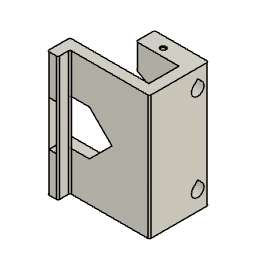
Ryobi PCL424 Cordless Trim Router Adjustable Fence (Autodesk Fusion 360 design; units mm, degrees)
Autodesk Fusion 360 part; units mm, degrees
sketch "Sketch1" plane through (0, 0, 0) normal (1, 0, 0) x (0, 1, 0)
  line L0 (0, 0) -> (29.2, 0) construction
  circle A0 centre (29.2, 0) radius 4.2
  line L1 (0, 2.5) -> (0, 20) construction
  circle A1 centre (-29.2, 0) radius 4.2
  line L2 (-29.2, 0) -> (-29.2, -4.2) construction
  line L3 (36.4, -5.2) -> (36.4, 7.2)
  line L4 (-36.4, -5.2) -> (-36.4, 7.2)
  line L5 (36.4, -5.2) -> (-36.4, -5.2)
  line L6 (36.4, 7.2) -> (-36.4, 7.2)
  line L7 (29.2, 0) -> (29.2, -4.2) construction
  line L8 (29.2, 0) -> (33.4, 0) construction
  line L9 (29.2, 0) -> (29.2, 4.2) construction
  dimension "d1" = 8.4
  dimension "d2" = 58.4
  dimension "d5" = 1
  dimension "d7" = 3
  dimension "d8" = 3
  constraint coincident L0.start origin
  constraint horizontal L0
  constraint coincident L0.end A0.centre
  constraint symmetric A0 L1 A1
  constraint coincident A1.centre L2.start
  constraint coincident A1 L2.end
  constraint vertical L3
  constraint symmetric L1 L3.start L4.start
  constraint symmetric L1 L3.end L4.end
  constraint coincident A0 L7.end
  constraint perpendicular L0 L7
  constraint coincident A0 L8.end
  constraint perpendicular L7 L8
  constraint coincident A0 L9.end
  constraint perpendicular L8 L9
  measures "d1" diameter of A0
  measures "d2" distance of L0.end A1.centre
  measures "d5" distance of L5 L7.end
  measures "d7" distance of L3 L8.end
  measures "d8" distance of L6 L9.end
extrude "Extrude1" add sketch "Sketch1" along normal blind 36
sketch "Sketch2" plane through (0, 0, -5.2) normal (0, 0, -1) x (1, 0, 0)
  line L0 (0, 36.4) -> (0, -36.4)
  line L1 (0, -36.4) -> (36, -36.4)
  line L2 (36, -36.4) -> (36, 36.4)
  line L3 (36, 36.4) -> (0, 36.4)
  line L4 (0, 0) -> (36, 0) construction
  line L5 (0, 0) -> (-9, 0) construction
  arc A0 (0, -24.9249) -> (0, 24.9249) centre (-9, 0) ccw
  line L6 (0, 36.4) -> (36, 36.4)
  line L7 (0, -36.4) -> (0, 36.4)
  line L8 (36, -36.4) -> (36, 36.4)
  line L9 (0, -36.4) -> (36, -36.4)
  arc A1 (0, -37.9473) -> (0, 37.9473) centre (-9, 0) ccw
  line L10 (28.7, -9.9855) -> (28.7, -36.4)
  line L11 (28.7, 9.9855) -> (28.7, 36.4)
  line L12 (28.7, 9.9855) -> (28.7, -9.9855)
  dimension "d11" = 45
  dimension "d12" = 53
  dimension "d15" = 39
  dimension "d29" = 7.3
  constraint coincident L4.start L5.start
  constraint midpoint L2 L4.end
  constraint perpendicular L0 L5
  constraint coincident L5.end A0.centre
  constraint coincident L0 A0.end
  constraint coincident L0 A0.start
  constraint coincident L7 A1.start
  constraint coincident L7 A1.end
  constraint coincident A1 L10.start
  constraint symmetric L4 L10.start L11.start
  constraint coincident L9 L10.end
  constraint perpendicular L9 L10
  constraint coincident L6 L11.end
  constraint perpendicular L6 L11
  measures "d11" distance of L4.end L5.end
  measures "d12" diameter of A0
  measures "d15" radius of A1
  measures "d29" distance of L2.end L11.end
extrude "Extrude2" cut sketch "Sketch2" against normal up to surface (12.4 mm away) contours L0 A0 L7
extrude "Extrude3" add sketch "Sketch2" along normal blind 20 contours L1 L2 L3 L6 L8 L9 A1 L10 L11 | A1 L12
sketch "Sketch4" plane through (0, 0, -25.2) normal (0, 0, -1) x (1, 0, 0)
  line L0 (28.7, 36.4) -> (28.7, -36.4)
  line L1 (28.7, -36.4) -> (36, -36.4)
  line L2 (36, -36.4) -> (36, 36.4)
  line L3 (36, 36.4) -> (28.7, 36.4)
  line L4 (36, -36.4) -> (-24, -36.4)
  line L5 (-24, -36.4) -> (-24, 36.4)
  line L6 (-24, 36.4) -> (36, 36.4)
  line L7 (36, 36.4) -> (36, -36.4)
  dimension "d30" = 60
  constraint horizontal L4
  constraint vertical L5
  constraint horizontal L6
  constraint vertical L7
  constraint coincident L1.end L2.start
  measures "d30" distance of L1.end L4.end
extrude "Extrude5" add sketch "Sketch4" along normal blind 15
sketch "Sketch5" plane through (0, -36.4, 0) normal (0, -1, 0) x (1, 0, 0)
  line L0 (0, 7.2) -> (0, -5.2)
  line L1 (0, -5.2) -> (28.7, -5.2)
  line L2 (28.7, -5.2) -> (28.7, -25.2)
  line L3 (28.7, -25.2) -> (-24, -25.2)
  line L4 (-24, -25.2) -> (-24, -40.2)
  line L5 (-24, -40.2) -> (36, -40.2)
  line L6 (36, -40.2) -> (36, 7.2)
  line L7 (36, 7.2) -> (0, 7.2)
  line L8 (36, -40.2) -> (-17, -40.2)
  line L9 (-17, -40.2) -> (-17, -32.2)
  line L10 (-17, -32.2) -> (36, -32.2)
  line L11 (36, -32.2) -> (36, -40.2)
  dimension "d33" = 7
  dimension "d34" = 7
  constraint horizontal L8
  constraint vertical L9
  constraint horizontal L10
  constraint vertical L11
  constraint coincident L5.end L6.start
  measures "d33" distance of L3 L10
  measures "d34" distance of L4 L9
extrude "Extrude6" cut sketch "Sketch5" against normal blind 72.8 contours L5 L6 L8 L9 L10 L11
sketch "Sketch6" plane through (0, 0, -32.2) normal (0, 0, -1) x (1, 0, 0)
  line L0 (36, 36.4) -> (-17, 36.4)
  line L1 (-17, 36.4) -> (-17, -36.4)
  line L2 (-17, -36.4) -> (36, -36.4)
  line L3 (36, -36.4) -> (36, 36.4)
  line L4 (-24, 36.4) -> (-24, -36.4)
  line L5 (-24, 15) -> (-4, 15)
  line L6 (-4, 15) -> (11, 0)
  line L7 (1.75, 0) -> (22.5, 0)
  line L8 (-4, -15) -> (11, 0)
  line L9 (-24, -15) -> (-4, -15)
  dimension "d37" = 30
  dimension "d38" = 35
  constraint coincident L4 L5.start
  constraint perpendicular L4 L5
  constraint symmetric L5.start L7 L9.start
  constraint symmetric L5.end L7 L8.start
  constraint symmetric L6.end L7 L8.end
  constraint perpendicular L6 L8
  constraint coincident L6.end L7
  measures "d37" distance of L5 L9
  measures "d38" distance of L4 L6.end
extrude "Extrude7" cut sketch "Sketch6" along normal blind 8 and the other way blind 7 contours L1 L5 L6 L8 L9 | L1 L4 L5 L9
move_face "OffsetFaces1" offset 5 2 faces at (21.5667, 36.4, 3.0667) (21.5667, -36.4, 3.0667)
sketch "Sketch7" plane through (0, 41.4, 0) normal (0, 1, 0) x (-1, 0, 0)
  line L0 (-36, -32.2) -> (17, -32.2)
  line L1 (17, -32.2) -> (17, -40.2)
  line L2 (17, -40.2) -> (24, -40.2)
  line L3 (24, -40.2) -> (24, -25.2)
  line L4 (24, -25.2) -> (-28.7, -25.2)
  line L5 (-28.7, -25.2) -> (-28.7, -5.2)
  line L6 (-28.7, -5.2) -> (0, -5.2)
  line L7 (0, -5.2) -> (0, 7.2)
  line L8 (0, 7.2) -> (-36, 7.2)
  line L9 (-36, 7.2) -> (-36, -32.2)
  circle A0 centre (-13, 0) radius 1.35
  line L10 (0, -4.2) -> (0, 4.2)
  line L11 (0, 0) -> (-13, 0) construction
  dimension "d44" = 2.7
  dimension "d47" = 13
  constraint coincident L11.start origin
  constraint coincident A0.centre L11.end
  constraint horizontal L11
  measures "d44" diameter of A0
  measures "d47" distance of L7 A0.centre
extrude "Extrude8" cut sketch "Sketch7" against normal blind 10 contours A0
mirror "Mirror1" about plane through (0, 0, 0) normal (0, 1, 0) of "Extrude8"
fillet "Fillet4" radius 1 14 edges at (36, 0, -32.2) (-17, -28.2, -32.2) (-17, -28.2, -40.2) (-17, 28.2, -32.2) (-17, 28.2, -40.2) (36, 0, 7.2) (0, -33.1624, 7.2) (0, 33.1624, 7.2) (0, 33.1624, -5.2) (0, -33.1624, -5.2) (-24, -28.2, -40.2) (-24, 28.2, -40.2) (-24, 28.2, -25.2) (-24, -28.2, -25.2)
sketch "Support Material" plane through (0, -15, 0) normal (0, 1, 0) x (-1, 0, 0)
  arc A0 (24, -26.2) -> (23, -25.2) centre (23, -26.2) ccw
  line L0 (23, -25.2) -> (4, -25.2)
  line L1 (4, -25.2) -> (4, -32.2)
  line L2 (4, -32.2) -> (16, -32.2)
  arc A1 (17, -33.2) -> (16, -32.2) centre (16, -33.2) ccw
  line L3 (17, -33.2) -> (17, -39.2)
  arc A2 (17, -39.2) -> (18, -40.2) centre (18, -39.2) ccw
  line L4 (18, -40.2) -> (23, -40.2)
  arc A3 (23, -40.2) -> (24, -39.2) centre (23, -39.2) ccw
  line L5 (24, -39.2) -> (24, -26.2)
  circle A4 centre (-13, 0) radius 1.35
  arc A5 (24, -26.2) -> (23, -25.2) centre (23, -26.2) ccw
  line L6 (24, -26.2) -> (24, -39.2)
  arc A6 (23, -40.2) -> (24, -39.2) centre (23, -39.2) ccw
  line L7 (23, -40.2) -> (18, -40.2)
  arc A7 (17, -39.2) -> (18, -40.2) centre (18, -39.2) ccw
  line L8 (17, -39.2) -> (17, -33.2)
  arc A8 (17, -33.2) -> (16, -32.2) centre (16, -33.2) ccw
  line L9 (16, -32.2) -> (-35, -32.2)
  arc A9 (-36, -31.2) -> (-35, -32.2) centre (-35, -31.2) ccw
  line L10 (-36, -31.2) -> (-36, 6.2)
  arc A10 (-35, 7.2) -> (-36, 6.2) centre (-35, 6.2) ccw
  line L11 (-35, 7.2) -> (-1, 7.2)
  arc A11 (0, 6.2) -> (-1, 7.2) centre (-1, 6.2) ccw
  line L12 (0, 6.2) -> (0, -4.2)
  arc A12 (-1, -5.2) -> (0, -4.2) centre (-1, -4.2) ccw
  line L13 (-1, -5.2) -> (-28.7, -5.2)
  line L14 (-28.7, -5.2) -> (-28.7, -25.2)
  line L15 (-28.7, -25.2) -> (23, -25.2)
  line L16 (18, -40.2) -> (18, -32.2)
  line L17 (18, -32.2) -> (16, -32.2)
  line L18 (23, -40.2) -> (22.7011, -40.2)
  line L19 (23, -25.2) -> (23, -40.2)
  constraint coincident A2.end L4.start
  constraint perpendicular L2 L16
  constraint coincident L2.end A1.end
  constraint tangent A8 L17
  constraint coincident L4.end A3.start
  constraint coincident L4 L18.end
  constraint parallel L4 L18
  constraint coincident A0.end L0.start
extrude "Extrude9" add sketch "Support Material" along normal blind 30 contours A0 A3 L5 A5 L6 A6 L19 | A1 L3 A2 A7 L8 A8 L16 L17
chamfer "Chamfer1" distance 0.5 angle 45 2 edges at (14.2586, -41.4, -0.4882) (14.2586, 41.4, 0.4882)
sketch "Make Holes 3d printable" plane through (0, 0, 0) normal (-1, 0, 0) x (0, -1, 0)
  line L0 (-29.2, -4.2) -> (-24.9249, -4.2)
  line L1 (-24.9249, -4.2) -> (-24.9249, 6.2)
  line L2 (-24.9249, 6.2) -> (-41.4, 6.2)
  line L3 (-41.4, 6.2) -> (-41.4, -4.2)
  line L4 (-41.4, -4.2) -> (-29.2, -4.2)
  circle A0 centre (-29.2, 0) radius 4.2
  circle A1 centre (-29.2, 0) radius 4.2
  circle A2 centre (29.2, 0) radius 4.2
  line L5 (29.2, 0) -> (-29.2, 0) construction
  line L6 (32.1698, 2.9698) -> (35.1397, 0)
  line L7 (-23.2603, 0) -> (-26.2302, 2.9698)
  line L8 (-23.2603, 0) -> (-26.2302, -2.9698)
  line L9 (32.1698, -2.9698) -> (35.1397, 0)
  constraint coincident A2.centre L5.start
  constraint coincident A0.centre A1.centre
  constraint coincident A2 L6.start
  constraint coincident L5 L7.start
  constraint coincident A1 L7.end
  constraint tangent A1 L7
  constraint symmetric L5 L6.start L9.start
  constraint symmetric L5 L6.end L9.end
  constraint symmetric L5 L7.start L8.start
  constraint symmetric L5 L7.end L8.end
  constraint perpendicular L7 L8
  constraint perpendicular L6 L9
  constraint coincident L6.end L9.end
  constraint tangent A2 L6
extrude "Extrude10" cut sketch "Make Holes 3d printable" against normal blind 36 contours L1 A0 A1 L7 L8 | L1 L7 L8 | A2 L6 L9
move_body "Move1" bodies 1 to x (1, 0, 0) y (0, 0, -1) z (0, 1, 0) at (0, -1, 1)
equation "d8 = d7"
equation "d34 = d33"
named bodies: "Ryobi router base fence"
